Autodesk Inventor part; units mm, degrees
(part 3 of 3)
sketch "Sketch23" plane through (0, 0, 0.6) normal (0, 0, 1) x (1, 0, 0)
  line L0 (2.2042, 2.4689) -> (2.8094, 2.4689)
  line L1 (2.8094, 2.4689) -> (2.8094, 2.1871)
  line L2 (2.8094, 2.1871) -> (2.2042, 2.1871)
  line L3 (2.2042, 2.1871) -> (2.2042, 2.4689)
  line L4 (2.6754, 2.4771) -> (2.8171, 2.4771)
  line L5 (2.8171, 2.4771) -> (2.8171, 2.1793)
  line L6 (2.8171, 2.1793) -> (2.6754, 2.1793)
  line L7 (2.6754, 2.1793) -> (2.6754, 2.4771)
  line L8 (2.1951, 2.4781) -> (2.3368, 2.4781)
  line L9 (2.3368, 2.4781) -> (2.3368, 2.1793)
  line L10 (2.3368, 2.1793) -> (2.1951, 2.1793)
  line L11 (2.1951, 2.1793) -> (2.1951, 2.4781)
  line L12 (5.7395, 2.5355) -> (5.7395, 1.9303)
  line L13 (5.7395, 1.9303) -> (5.4577, 1.9303)
  line L14 (5.4577, 1.9303) -> (5.4577, 2.5355)
  line L15 (5.4577, 2.5355) -> (5.7395, 2.5355)
  line L16 (5.7477, 2.0643) -> (5.7477, 1.9226)
  line L17 (5.7477, 1.9226) -> (5.4499, 1.9226)
  line L18 (5.4499, 1.9226) -> (5.4499, 2.0643)
  line L19 (5.4499, 2.0643) -> (5.7477, 2.0643)
  line L20 (5.7487, 2.5446) -> (5.7487, 2.4029)
  line L21 (5.4499, 2.5446) -> (5.7487, 2.5446)
  line L22 (5.4499, 2.4029) -> (5.4499, 2.5446)
  line L23 (5.7487, 2.4029) -> (5.4499, 2.4029)
  line L24 (6.343, 2.5355) -> (6.343, 1.9303)
  line L25 (6.343, 1.9303) -> (6.0612, 1.9303)
  line L26 (6.0612, 1.9303) -> (6.0612, 2.5355)
  line L27 (6.0612, 2.5355) -> (6.343, 2.5355)
  line L28 (6.3512, 2.0643) -> (6.3512, 1.9226)
  line L29 (6.3512, 1.9226) -> (6.0535, 1.9226)
  line L30 (6.0535, 1.9226) -> (6.0535, 2.0643)
  line L31 (6.0535, 2.0643) -> (6.3512, 2.0643)
  line L32 (6.3522, 2.5446) -> (6.3522, 2.4029)
  line L33 (6.0535, 2.5446) -> (6.3522, 2.5446)
  line L34 (6.0535, 2.4029) -> (6.0535, 2.5446)
  line L35 (6.3522, 2.4029) -> (6.0535, 2.4029)
  line L36 (3.8837, -2.4133) -> (3.8837, -3.0185)
  line L37 (3.8837, -3.0185) -> (3.6018, -3.0185)
  line L38 (3.6018, -3.0185) -> (3.6018, -2.4133)
  line L39 (3.6018, -2.4133) -> (3.8837, -2.4133)
  line L40 (3.8919, -2.8845) -> (3.8919, -3.0262)
  line L41 (3.8919, -3.0262) -> (3.5941, -3.0262)
  line L42 (3.5941, -3.0262) -> (3.5941, -2.8845)
  line L43 (3.5941, -2.8845) -> (3.8919, -2.8845)
  line L44 (3.8929, -2.4042) -> (3.8929, -2.5459)
  line L45 (3.5941, -2.4042) -> (3.8929, -2.4042)
  line L46 (3.5941, -2.5459) -> (3.5941, -2.4042)
  line L47 (3.8929, -2.5459) -> (3.5941, -2.5459)
  line L48 (6.5014, -3.1149) -> (6.5014, -3.7201)
  line L49 (6.5014, -3.7201) -> (6.2196, -3.7201)
  line L50 (6.2196, -3.7201) -> (6.2196, -3.1149)
  line L51 (6.2196, -3.1149) -> (6.5014, -3.1149)
  line L52 (6.5096, -3.5861) -> (6.5096, -3.7278)
  line L53 (6.5096, -3.7278) -> (6.2119, -3.7278)
  line L54 (6.2119, -3.7278) -> (6.2119, -3.5861)
  line L55 (6.2119, -3.5861) -> (6.5096, -3.5861)
  line L56 (6.5106, -3.1058) -> (6.5106, -3.2475)
  line L57 (6.2119, -3.1058) -> (6.5106, -3.1058)
  line L58 (6.2119, -3.2475) -> (6.2119, -3.1058)
  line L59 (6.5106, -3.2475) -> (6.2119, -3.2475)
  line L60 (4.5388, 2.7584) -> (5.144, 2.7584)
  line L61 (5.144, 2.7584) -> (5.144, 2.4766)
  line L62 (5.144, 2.4766) -> (4.5388, 2.4766)
  line L63 (4.5388, 2.4766) -> (4.5388, 2.7584)
  line L64 (5.01, 2.7666) -> (5.1517, 2.7666)
  line L65 (5.1517, 2.7666) -> (5.1517, 2.4689)
  line L66 (5.1517, 2.4689) -> (5.01, 2.4689)
  line L67 (5.01, 2.4689) -> (5.01, 2.7666)
  line L68 (4.5297, 2.7676) -> (4.6714, 2.7676)
  line L69 (4.5297, 2.4689) -> (4.5297, 2.7676)
  line L70 (4.6714, 2.4689) -> (4.5297, 2.4689)
  line L71 (4.6714, 2.7676) -> (4.6714, 2.4689)
  line L72 (3.6184, 2.7584) -> (4.2236, 2.7584)
  line L73 (4.2236, 2.7584) -> (4.2236, 2.4766)
  line L74 (4.2236, 2.4766) -> (3.6184, 2.4766)
  line L75 (3.6184, 2.4766) -> (3.6184, 2.7584)
  line L76 (4.0897, 2.7666) -> (4.2314, 2.7666)
  line L77 (4.2314, 2.7666) -> (4.2314, 2.4689)
  line L78 (4.2314, 2.4689) -> (4.0897, 2.4689)
  line L79 (4.0897, 2.4689) -> (4.0897, 2.7666)
  line L80 (3.6093, 2.7676) -> (3.751, 2.7676)
  line L81 (3.6093, 2.4689) -> (3.6093, 2.7676)
  line L82 (3.751, 2.4689) -> (3.6093, 2.4689)
  line L83 (3.751, 2.7676) -> (3.751, 2.4689)
  line L84 (4.5311, 2.1669) -> (5.1363, 2.1669)
  line L85 (5.1363, 2.1669) -> (5.1363, 1.8851)
  line L86 (5.1363, 1.8851) -> (4.5311, 1.8851)
  line L87 (4.5311, 1.8851) -> (4.5311, 2.1669)
  line L88 (5.0023, 2.1751) -> (5.144, 2.1751)
  line L89 (5.144, 2.1751) -> (5.144, 1.8774)
  line L90 (5.144, 1.8774) -> (5.0023, 1.8774)
  line L91 (5.0023, 1.8774) -> (5.0023, 2.1751)
  line L92 (4.522, 2.1761) -> (4.6637, 2.1761)
  line L93 (4.522, 1.8774) -> (4.522, 2.1761)
  line L94 (4.6637, 1.8774) -> (4.522, 1.8774)
  line L95 (4.6637, 2.1761) -> (4.6637, 1.8774)
  point P0 (0, 0)
  constraints: 192 end point, 48 parallel, 24 perpendicular, 12 horizontal
extrude "Extrusion32" add sketch "Sketch22" along normal blind 0.58 contours L0 L1 L6 L3 | L6 L1 L8 L3 | L8 L1 L2 L3
extrude "Extrusion31" add sketch "Sketch22" along normal blind 0.6 contours L3 L6 L7 L4 L5 L1 L0 | L0 L1 L6 L3 | L8 L1 L2 L3 | L3 L2 L1 L8 L9 L10 L11
extrude "Extrusion33" add sketch "Sketch23" along normal blind 0.2 contours L3 L2 L9 L10 L11 L8 L0 | L0 L9 L2 L3 | L7 L4 L5 L6 L2 L1 L0 | L0 L1 L2 L7 | L15 L14 L23 L22 L21 L20 L12 | L12 L23 L14 L15 | L19 L16 L17 L18 L14 L13 L12 | L12 L13 L14 L19 | L27 L26 L35 L34 L33 L32 L24 | L24 L35 L26 L27 | L31 L28 L29 L30 L26 L25 L24 | L24 L25 L26 L31 | L39 L38 L47 L46 L45 L44 L36 | L36 L47 L38 L39 | L43 L40 L41 L42 L38 L37 L36 | L36 L37 L38 L43 | L51 L50 L59 L58 L57 L56 L48 | L48 L59 L50 L51 | L55 L52 L53 L54 L50 L49 L48 | L48 L49 L50 L55 | L63 L62 L71 L70 L69 L68 L60 | L60 L71 L62 L63 | L67 L64 L65 L66 L62 L61 L60 | L60 L61 L62 L67 | L75 L74 L83 L82 L81 L80 L72 | L72 L83 L74 L75 | L79 L76 L77 L78 L74 L73 L72 | L72 L73 L74 L79 | L87 L86 L95 L94 L93 L92 L84 | L84 L95 L86 L87 | L91 L88 L89 L90 L86 L85 L84 | L84 L85 L86 L91
extrude "Extrusion34" add sketch "Sketch23" along normal blind 0.19 contours L0 L9 L2 L3 | L0 L7 L2 L9 | L0 L1 L2 L7 | L12 L23 L14 L15 | L12 L19 L14 L23 | L12 L13 L14 L19 | L24 L35 L26 L27 | L24 L31 L26 L35 | L24 L25 L26 L31 | L36 L47 L38 L39 | L36 L43 L38 L47 | L36 L37 L38 L43 | L48 L59 L50 L51 | L48 L55 L50 L59 | L48 L49 L50 L55 | L60 L71 L62 L63 | L60 L67 L62 L71 | L60 L61 L62 L67
extrude "Extrusion35" add sketch "Sketch23" along normal blind 0.19 contours L72 L83 L74 L75 | L72 L79 L74 L83 | L72 L73 L74 L79 | L84 L95 L86 L87 | L84 L91 L86 L95 | L84 L85 L86 L91
sketch "Sketch24" plane through (0, 0, 0.6) normal (0, 0, 1) x (1, 0, 0)
  line L0 (3.2103, 2.8793) -> (2.1423, 2.8793)
  line L1 (2.1423, 2.8793) -> (2.1423, 3.8)
  line L2 (2.1423, 3.8) -> (3.2103, 3.8)
  line L3 (3.2103, 3.8) -> (3.2103, 2.8793)
  line L4 (3.5476, 3.8349) -> (4.6655, 3.8349)
  line L5 (4.6655, 3.8349) -> (4.6655, 3.1353)
  line L6 (4.6655, 3.1353) -> (3.5476, 3.1353)
  line L7 (3.5476, 3.1353) -> (3.5476, 3.8349)
  line L8 (5.4338, 3.9785) -> (6.558, 3.9785)
  line L9 (6.558, 3.9785) -> (6.558, 3.0479)
  line L10 (6.558, 3.0479) -> (5.4338, 3.0479)
  line L11 (5.4338, 3.0479) -> (5.4338, 3.9785)
  point P0 (0, 0)
  constraints: 24 end point, 6 parallel, 3 horizontal, 3 perpendicular
extrude "Extrusion36" add sketch "Sketch24" along normal blind 0.4 contours L0 L1 L2 L3
extrude "Extrusion37" add sketch "Sketch24" along normal blind 0.3 contours L4 L5 L6 L7
extrude "Extrusion38" add sketch "Sketch24" along normal blind 0.5 contours L8 L9 L10 L11
sketch "Sketch25" plane through (0, 0, 0.6) normal (0, 0, 1) x (1, 0, 0)
  line L0 (6.5094, -4.2989) -> (6.5094, -3.6559)
  line L1 (6.169, -3.6559) -> (6.169, -3.9785)
  line L2 (6.169, -3.6559) -> (6.5094, -3.6559)
  line L3 (3.5941, -3.0622) -> (3.5941, -2.724)
  line L4 (3.5941, -2.724) -> (6.1692, -2.724)
  line L5 (6.1692, -2.724) -> (6.1692, -2.2391)
  line L6 (6.1692, -3.2475) -> (6.1692, -3.0622)
  line L7 (6.1692, -3.0622) -> (3.5941, -3.0622)
  line L8 (3.6093, -2.4787) -> (3.9118, -2.4787)
  line L9 (3.9118, -2.4787) -> (3.9118, 0.8709)
  line L10 (6.1394, 1.4052) -> (5.7477, 1.4052)
  line L11 (5.4577, 1.4052) -> (4.8939, 1.4052)
  line L12 (4.5837, 2.3493) -> (3.2242, 2.3493)
  line L13 (3.0052, 2.678) -> (3.5236, 3.4197)
  line L14 (4.3947, 3.2) -> (5.3072, 3.2)
  line L15 (5.3072, 3.2) -> (4.9971, 2.7564)
  line L16 (1.0643, 4.3) -> (1.0643, 1.7512)
  line L17 (1.0643, 1.7512) -> (4.5307, 1.7512)
  line L18 (4.5307, 1.7512) -> (4.5307, 1.4052)
  line L19 (4.5307, 1.4052) -> (3.8093, 1.4052)
  line L20 (3.6093, 1.2052) -> (3.6093, -2.4787)
  line L21 (4.1118, 1.0709) -> (6.3394, 1.0709)
  line L22 (6.3394, 1.2052) -> (6.3394, 1.0709)
  line L23 (6.1692, -2.2391) -> (6.5096, -2.2391)
  line L24 (6.5096, -2.2391) -> (6.5096, -3.2475)
  line L25 (6.5096, -3.2475) -> (6.1692, -3.2475)
  line L26 (6.5094, -4.2989) -> (1.3668, -4.2989)
  line L27 (1.3668, -4.2989) -> (1.3668, -3.9785)
  line L28 (1.3668, -3.9785) -> (6.169, -3.9785)
  line L29 (1.0643, 4.3) -> (2.5, 4.3)
  line L30 (2.5, 4.3) -> (2.5, 3.1062)
  line L31 (2.5, 3.1062) -> (3.0343, 3.1062)
  line L32 (3.0343, 3.1062) -> (3.0343, 4.508)
  line L33 (3.0343, 4.508) -> (3.1773, 4.7126)
  line L34 (3.1773, 4.7126) -> (3.1773, 3.2643)
  line L35 (3.1773, 3.2643) -> (3.418, 3.6823)
  line L36 (3.418, 3.6823) -> (3.418, 3.9758)
  line L37 (3.418, 3.9758) -> (4.0312, 3.9758)
  line L38 (4.0312, 3.9758) -> (4.0312, 4.4962)
  line L39 (4.0312, 4.4962) -> (4.1708, 4.7386)
  line L40 (4.1708, 4.7386) -> (4.1708, 3.9758)
  line L41 (3.0052, 2.678) -> (3.0052, 2.3493)
  line L42 (3.0052, 2.3493) -> (3.2242, 2.3493)
  line L43 (3.5236, 3.4197) -> (4.2926, 3.4197)
  line L44 (4.2926, 3.4197) -> (3.8161, 2.6969)
  line L45 (3.8161, 2.6969) -> (4.07, 2.6969)
  line L46 (4.07, 2.6969) -> (4.3947, 3.2)
  line L47 (4.5837, 2.3493) -> (4.5837, 2.747)
  line L48 (4.5837, 2.747) -> (4.8939, 2.747)
  line L49 (4.8939, 2.747) -> (4.8939, 1.4052)
  line L50 (5.4577, 1.4052) -> (5.4577, 2.1579)
  line L51 (5.4577, 2.1579) -> (5.7477, 2.1579)
  line L52 (5.7477, 2.1579) -> (5.7477, 1.4052)
  line L53 (5.4577, 2.3861) -> (5.4577, 2.5564)
  line L54 (5.6577, 2.7564) -> (5.9781, 2.7564)
  line L55 (6.1781, 2.9564) -> (6.1781, 3.2)
  line L56 (4.9971, 2.7564) -> (4.9971, 2.455)
  line L57 (4.9971, 2.455) -> (5.0663, 2.455)
  line L58 (5.0663, 2.455) -> (5.5842, 3.2)
  line L59 (5.5842, 3.2) -> (6.1781, 3.2)
  line L60 (5.4577, 2.3861) -> (5.7477, 2.3861)
  line L61 (5.7477, 2.3861) -> (5.7477, 2.4605)
  line L62 (5.7477, 2.4605) -> (6.3402, 2.4605)
  line L63 (6.5402, 2.6605) -> (6.5402, 3.9758)
  line L64 (6.5402, 3.9758) -> (4.1708, 3.9758)
  arc A0 (5.9781, 2.7564) -> (6.1781, 2.9564) centre (5.9781, 2.9564) ccw
  arc A1 (5.6577, 2.7564) -> (5.4577, 2.5564) centre (5.6577, 2.5564) ccw
  arc A2 (6.3402, 2.4605) -> (6.5402, 2.6605) centre (6.3402, 2.6605) ccw
  arc A3 (6.3394, 1.2052) -> (6.1394, 1.4052) centre (6.1394, 1.2052) ccw
  arc A4 (3.8093, 1.4052) -> (3.6093, 1.2052) centre (3.8093, 1.2052) ccw
  arc A5 (4.1118, 1.0709) -> (3.9118, 0.8709) centre (4.1118, 0.8709) ccw
  point P0 (0, 0)
  point P1 (1.6, -4.3)
  point P2 (6.6526, -2.2391)
  point P3 (4.8939, -2.2391)
  point P4 (3.6093, 1.4052)
  point P5 (5.4577, 2.7564)
  dimension "d1204" = 0.2
  constraints: 130 end point, 23 perpendicular, 14 point on line, 12 point on circle, 12 tangent, 8 horizontal, 8 parallel, 7 vertical, 6 centre point, 5 equal radius
  measures "d1204" radius of A0
extrude "Extrusion39" add sketch "Sketch25" along normal blind 0.01
sketch "Sketch27" plane through (0, 0, 0) normal (0, 0, -1) x (-1, 0, 0)
  line L0 (6.762, -3.6976) -> (-2.3571, -3.6976)
  line L1 (-2.3571, -3.6976) -> (-2.3571, -4.039)
  line L2 (-6.7512, -4.039) -> (-6.7512, -3.685)
  line L3 (-6.7512, -3.685) -> (-2.6333, -3.685)
  line L4 (-2.6333, -3.685) -> (-2.6333, -3.4266)
  line L5 (-2.6333, -3.4266) -> (-2.0924, -3.4266)
  line L6 (-2.0924, -3.4266) -> (-2.0924, 2.4929)
  line L7 (-2.0924, 2.4929) -> (-6.7512, 2.4929)
  line L8 (-6.7512, 2.4929) -> (-6.7512, 4.3064)
  line L9 (-6.7512, 4.3064) -> (-4.5056, 4.3064)
  line L10 (-4.5056, 4.3064) -> (-4.5056, 3.6612)
  line L11 (-4.5056, 3.6612) -> (-2.0924, 3.6612)
  line L12 (-2.0924, 3.6612) -> (-2.0924, 3.9764)
  line L13 (-2.0924, 3.9764) -> (-1.5075, 3.9764)
  line L14 (-1.5075, 3.9764) -> (-1.5075, 3.6612)
  line L15 (-1.5075, 3.6612) -> (-1.0828, 3.6612)
  line L16 (6.762, 3.6764) -> (6.762, 2.6605)
  line L17 (6.762, 2.6605) -> (5.8498, 2.6605)
  line L18 (5.8498, 2.6605) -> (5.8498, -2.6879)
  line L19 (5.8498, -2.6879) -> (6.762, -2.6879)
  line L20 (6.762, -2.6879) -> (6.762, -3.6976)
  line L21 (6.762, 3.6764) -> (2.5, 3.6764)
  line L22 (1.9028, 3.6764) -> (1.5, 3.6764)
  line L23 (2.5, 3.6764) -> (2.5, 3.9664)
  line L24 (2.5, 3.9664) -> (1.9028, 3.9664)
  line L25 (1.9028, 3.9664) -> (1.9028, 3.6764)
  line L26 (1.5, 3.6764) -> (1.5, 3.9664)
  line L27 (1.5, 3.9664) -> (0.9104, 3.9664)
  line L28 (0.9104, 3.9664) -> (0.9104, 3.6777)
  line L29 (0.9104, 3.6777) -> (-0.5068, 3.6777)
  line L30 (-0.5068, 3.6777) -> (-0.5068, 3.9664)
  line L31 (-0.5068, 3.9664) -> (-1.0828, 3.9664)
  line L32 (-1.0828, 3.9664) -> (-1.0828, 3.6612)
  line L33 (-2.3571, -4.039) -> (-6.7512, -4.039)
  point P0 (0, 0)
  point P1 (1.9, 3.8)
  point P2 (2.5, 3.8)
  constraints: 70 end point, 18 perpendicular, 14 point on line, 2 horizontal, 2 vertical, 1 parallel
extrude "Extrusion40" add sketch "Sketch27" along normal blind 0.008
sketch "Sketch28" plane through (0, 0, -0.008) normal (0, 0, -1) x (-1, 0, 0)
  line L0 (5.9242, -3.0907) -> (6.3975, -3.0907)
  line L1 (6.3975, -3.0907) -> (6.1608, -3.5006)
  line L2 (6.1608, -3.5006) -> (5.9242, -3.0907)
  line L3 (6.5, -3.8) -> (5.9, -3.8) projected
  point P0 (0, 0)
  point P1 (6.1608, -3.2273)
  constraints: 6 end point, 1 parallel, 7 other
extrude "Extrusion41" add sketch "Sketch28" along normal blind 0.001
